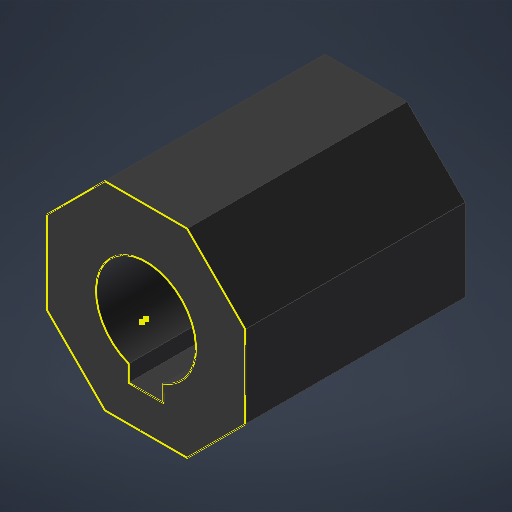
# Autodesk Inventor part: spool_keyway
Saved by Autodesk Inventor 2026.1 (Build 301233000, 233)
## iProperties
Created: 2026-04-16
Part Number: spool_keyway
Material: Generic
Document SubType Name: Modeling
Designer: aaron
Density: 1 g/cm^3
Appearance: Default
Author: aaron
Autodesk Inventor part; units mm, degrees
ref_plane "YZ Plane" through (0, 0, 0) normal (1, 0, 0) x (0, 1, 0)
ref_plane "XZ Plane" through (0, 0, 0) normal (0, 1, 0) x (-1, 0, 0)
ref_plane "XY Plane" through (0, 0, 0) normal (0, 0, 1) x (1, 0, 0)
sketch "Sketch1" plane through (0, 0, 0) normal (0, 0, 1) x (1, 0, 0)
  circle A0 centre (-19.4529, 0.6357) radius 3.1
  circle A1 centre (0.5471, -19.3643) radius 3.1
  circle A2 centre (20.5471, 0.6357) radius 3.1
  circle A3 centre (-13.595, 14.7778) radius 3.1
  line L0 (15.4871, -5.5527) -> (6.7355, -14.3043)
  line L1 (6.7355, -14.3043) -> (-5.6412, -14.3043)
  line L2 (-5.6412, -14.3043) -> (-14.3929, -5.5527)
  line L3 (-14.3929, -5.5527) -> (-14.3929, 6.824)
  line L4 (-14.3929, 6.824) -> (-5.6412, 15.5757)
  line L5 (-5.6412, 15.5757) -> (6.7355, 15.5757)
  line L6 (6.7355, 15.5757) -> (15.4871, 6.824)
  line L7 (15.4871, 6.824) -> (15.4871, -5.5527)
  circle A4 centre (14.6893, 14.7778) radius 3.1
  circle A5 centre (14.6893, -13.5064) radius 3.1
  circle A6 centre (-13.595, -13.5064) radius 3.1
  arc A7 (-10.3042, 22.9357) -> (11.3984, 22.9357) centre (0.5471, 0.6357) ccw
  line L8 (-10.3042, 22.9357) -> (11.3984, 22.9357)
  point P0 (0, 0)
  constraints: 18 end point, 8 centre point, 2 point on circle
extrude "Extrusion1" add sketch "Sketch1" along normal blind 33 contours L0 L1 L2 L3 L4 L5 L6 L7
sketch "Sketch2" plane through (0, 0, 33) normal (0, 0, 1) x (1, 0, 0)
  arc A0 (3.1471, -6.3992) -> (-2.0529, -6.3992) centre (0.5471, 0.6357) ccw
  line L0 (3.1471, -8.8943) -> (3.1471, -6.3992)
  line L1 (-2.0529, -8.8943) -> (3.1471, -8.8943)
  line L2 (-2.0529, -8.8943) -> (-2.0529, -6.3992)
  line L3 (0.5471, 0.6357) -> (-14.3929, 0.6357)
  line L4 (-14.3929, 6.824) -> (-14.3929, -5.5527) projected
  line L5 (0.5471, 0.6357) -> (15.4871, 0.6357)
  line L6 (15.4871, -5.5527) -> (15.4871, 6.824) projected
  line L7 (0.5471, 0.6357) -> (0.5471, 15.5757)
  line L8 (6.7355, 15.5757) -> (-5.6412, 15.5757) projected
  point P0 (0, 0)
  point P1 (0.5471, 0.6357)
  point P2 (1.7246, 0.9714)
  dimension "d2" = 7.5
  dimension "d3" = 5.2
  dimension "d4" = 2.4951
  dimension "d5" = 2.6
  constraints: 12 end point, 3 midpoint, 2 equal length, 2 point on circle, 1 centre point, 1 horizontal, 1 perpendicular, 1 point on line
  measures "d2" radius of A0
  measures "d3" distance of L1.start L0.start
  measures "d4" distance of L0.start L0.end
  measures "d5" distance from line of point (0.547, 0.636) L0
extrude "Extrusion2" cut sketch "Sketch2" against normal through all
thicken "Thicken1" operation cut thickness 0.05 both sides no extend neighbours no toward (0, -1, 0) faces at (2.6099, 15.5757, 11) (12.5699, 9.7413, 22) (15.4871, -1.4271, 11) (9.6527, -11.3871, 11) (-1.5157, -14.3043, 11) (-11.4757, -8.4699, 11) (-14.3929, 2.6985, 11) (-8.5585, 12.6585, 11)
sketch "Sketch3" plane through (0, 0, 33) normal (0, 0, 1) x (1, 0, 0)
  line L0 (6.7148, -14.2543) -> (15.4371, -5.5319) projected
  line L1 (15.4371, -5.5319) -> (15.4371, 6.8033) projected
  line L2 (15.4371, 6.8033) -> (6.7148, 15.5257) projected
  line L3 (6.7148, 15.5257) -> (-5.6205, 15.5257) projected
  line L4 (-5.6205, 15.5257) -> (-14.3429, 6.8033) projected
  line L5 (-14.3429, 6.8033) -> (-14.3429, -5.5319) projected
  line L6 (-14.3429, -5.5319) -> (-5.6205, -14.2543) projected
  line L7 (-5.6205, -14.2543) -> (6.7148, -14.2543) projected
  line L8 (-2.0529, -8.8943) -> (-2.0529, -6.3992) projected
  arc A0 (3.1471, -6.3992) -> (-2.0529, -6.3992) centre (0.5471, 0.6357) ccw projected
  line L9 (3.1471, -6.3992) -> (3.1471, -8.8943) projected
  line L10 (3.1471, -8.8943) -> (-2.0529, -8.8943) projected
  point P0 (0, 0)
body "Solid1"
